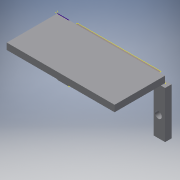
# Autodesk Inventor part: Servo_vice
Saved by Autodesk Inventor 2016 (Build 200138000, 138)
## iProperties
Created: 2015-10-07
Part Number: Servo_vice
Material: Generic
Document SubType Name: Modeling
Designer: powasar16
Density: 1 g/cm^3
Appearance: Default
Author: powasar16
Autodesk Inventor part; units mm, degrees
ref_plane "YZ Plane" through (0, 0, 0) normal (1, 0, 0) x (0, 1, 0)
ref_plane "XZ Plane" through (0, 0, 0) normal (0, 1, 0) x (-1, 0, 0)
ref_plane "XY Plane" through (0, 0, 0) normal (0, 0, 1) x (1, 0, 0)
sketch "Sketch1" plane through (0, 0, 0) normal (0, 0, 1) x (1, 0, 0)
  line L0 (-4.3, 0) -> (27.3, 0) projected
  line L1 (27.5, -0.2) -> (27.5, -5.5) projected
  line L2 (-4.3, -12) -> (27.3, -12) projected
  line L3 (27.5, -6.5) -> (27.5, -11.8) projected
  line L4 (-4.5, -0.2) -> (-4.5, -5.5) projected
  line L5 (-4.5, -6.5) -> (-4.5, -11.8) projected
  line L6 (-4.5, 0) -> (-1.071, 0)
  line L7 (-1.071, 0) -> (-1.071, -12)
  line L8 (-1.071, -12) -> (-4.5, -12)
  line L9 (-4.5, -12) -> (-4.5, 0)
  arc A0 (-3.366, -6.5) -> (-3.366, -5.5) centre (-2.5, -6) ccw projected
  circle A1 centre (-2.5, -6) radius 1
  line L10 (27.5, -12) -> (24.071, -12)
  line L11 (24.071, -12) -> (24.071, 0)
  line L12 (24.071, 0) -> (27.5, 0)
  line L13 (27.5, 0) -> (27.5, -12)
  arc A2 (26.366, -5.5) -> (26.366, -6.5) centre (25.5, -6) ccw projected
  circle A3 centre (25.5, -6) radius 1
  line L14 (-1.071, 0) -> (-4.5, 0)
  line L15 (-4.5, 0) -> (-4.5, 1.905)
  line L16 (-4.5, 1.905) -> (-1.071, 1.905)
  line L17 (-1.071, 1.905) -> (-1.071, 0)
  line L18 (11.5, 0) -> (11.5, -12) construction
  line L19 (27.5, 0) -> (24.071, 0)
  line L20 (24.071, 0) -> (27.5, 0)
  line L21 (27.5, 0) -> (27.5, 1.905)
  line L22 (27.5, 1.905) -> (24.071, 1.905)
  line L23 (24.071, 1.905) -> (24.071, 0)
  point P0 (0, 0)
  dimension "d0" = 3.429
  dimension "d1" = 3.429
  dimension "d2" = 1.905
  constraints: 36 end point, 6 parallel, 4 point on line, 4 symmetric about line, 3 collinear, 3 horizontal, 3 perpendicular, 2 coincident, 2 midpoint, 1 centre point, 1 concentric, 3 other
  measures "d0" distance between parallel lines of L7 L4
  measures "d1" distance between parallel lines of L1 L11
  measures "d2" distance between parallel lines of L0 L16
extrude "Extrusion1" add sketch "Sketch1" along normal blind 1.905 contours L6 L15 L16 L17 L0 | L0 L7 L2 L8 L9 L5 L4 L6 | L23 L22 L21 L12 L0 | L0 L12 L13 L1 L3 L10 L2 L11
ref_plane "Work Plane1" through (0, 3.175, 15) normal (0, 1, 0) x (1, 0, 0)
sketch "Sketch2" plane through (0, 3.175, 15) normal (0, 1, 0) x (1, 0, 0)
  line L0 (-1.071, 15) -> (-4.5, 15) projected
  line L1 (-4.5, 15) -> (-4.5, 13.095) projected
  line L2 (-1.071, 13.095) -> (-4.5, 13.095) projected
  line L3 (-1.071, 15) -> (-1.071, 13.095) projected
  line L4 (27.5, 15) -> (24.071, 15) projected
  line L5 (24.071, 15) -> (24.071, 13.095) projected
  line L6 (27.5, 13.095) -> (24.071, 13.095) projected
  line L7 (27.5, 15) -> (27.5, 13.095) projected
  line L8 (22.8, 0) -> (0.2, 0) projected
  line L9 (-4.5, 13.095) -> (27.5, 13.095)
  line L10 (27.5, 13.095) -> (27.5, -1.905)
  line L11 (27.5, -1.905) -> (-4.5, -1.905)
  line L12 (-4.5, -1.905) -> (-4.5, 13.095)
  point P0 (0, 15)
  dimension "d5" = 1.905
  constraints: 8 end point, 2 parallel, 1 collinear, 1 horizontal, 1 perpendicular
  measures "d5" distance between parallel lines of L8 L11
extrude "Extrusion2" add sketch "Sketch2" along normal blind 1.905 contours L9 L6 L10 L11 L12 L2
sketch "Sketch3" plane through (27.5, 3.175, 1.905) normal (0, 0, -1) x (-1, 0, 0)
  line L0 (28.571, -15.175) -> (28.571, -1.27) projected
  line L1 (0, 0) -> (32, 0) projected
  line L2 (28.571, 0) -> (32, 0)
  line L3 (32, 0) -> (32, 1.905)
  line L4 (32, 1.905) -> (28.571, 1.905)
  line L5 (28.571, 1.905) -> (28.571, 0)
  point P0 (27.5, -3.175)
  constraints: 8 end point, 2 parallel, 1 collinear, 1 horizontal, 1 perpendicular, 1 point on line
sketch "Sketch4" plane through (-4.5, 1.905, 0) normal (0, 1, 0) x (1, 0, 0)
  point P0 (4.5, 0)
body "Solid1"
